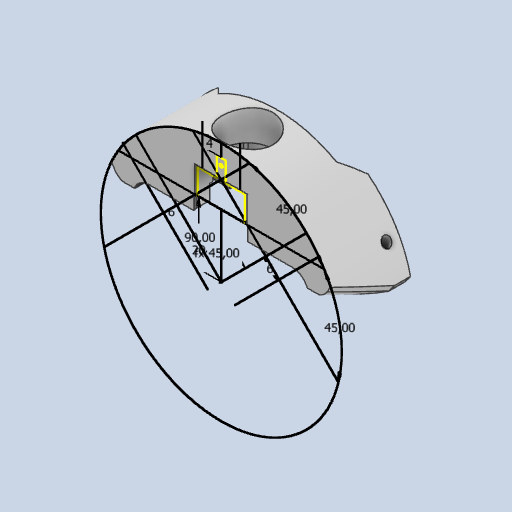
# Autodesk Inventor part: camera_disk
Saved by Autodesk Inventor 2023 (Build 270158000, 158)
## iProperties
Created: 2025-10-11
Part Number: camera_disk
Material: Типовые
Document SubType Name: Modeling
Designer: Andrey
Density: 1 g/cm^3
Appearance: По умолчанию
Author: Andrey
Autodesk Inventor part; units mm, degrees
ref_plane "YZ Plane" through (0, 0, 0) normal (1, 0, 0) x (0, 1, 0)
ref_plane "XZ Plane" through (0, 0, 0) normal (0, 1, 0) x (-1, 0, 0)
ref_plane "XY Plane" through (0, 0, 0) normal (0, 0, 1) x (1, 0, 0)
sketch "Эскиз1" plane through (0, 0, 0) normal (0, 0, 1) x (1, 0, 0)
  line L0 (-15, -8) -> (0, -8) projected
  line L1 (0, 0) -> (0, -8) projected
  line L2 (-6.1, 0) -> (0, 0) projected
  line L3 (-6.1, 0) -> (-6.1, 6.3) projected
  line L4 (-8.9, 6.3) -> (-6.1, 6.3) projected
  line L5 (-8.9, 0) -> (-8.9, 6.3) projected
  line L6 (-15, 0) -> (-8.9, 0) projected
  line L7 (-15, 0) -> (-15, -8) projected
  circle A0 centre (-7.5, 4.1) radius 0.5 projected
  line L8 (-1.5, 13.2534) -> (-1.5, 0.5534)
  line L9 (-13.5, 13.2534) -> (-13.5, 0.5534)
  circle A1 centre (-7.5, -28) radius 38.3
  line L10 (-7.5, -8) -> (-7.5, -28)
  line L11 (-7.5, 6.3) -> (-7.5, 10.3)
  line L12 (-7.5, -28) -> (-34.5822, -0.9178)
  line L13 (-7.5, -28) -> (19.5822, -0.9178)
  line L14 (-11.7426, -32.2426) -> (-38.8248, -5.1605)
  line L15 (-3.2574, -32.2426) -> (23.8248, -5.1605)
  line L16 (25.1633, -8) -> (-40.1633, -8)
  line L17 (1.4543, 9.2386) -> (-44.7386, -36.9543)
  line L18 (29.7386, -36.9543) -> (-16.4543, 9.2386)
  dimension "d0" = 4
  dimension "d1" = 20
  dimension "d2" = 90
  dimension "d3" = 45
  dimension "d4" = 6
  dimension "d5" = 6
  dimension "d13" = 45
  dimension "d17" = 45
  constraints: 22 end point, 5 point on circle, 4 vertical, 2 midpoint, 2 parallel, 1 centre point, 1 coincident, 1 collinear, 1 horizontal, 12 other
  measures "d0" distance of L11.start L11.end
  measures "d1" distance of L10.start L10.end
  measures "d2" angle of L12 L13
  measures "d3" angle of L10 L12
  measures "d4" distance between parallel lines of L12 L14
  measures "d5" distance between parallel lines of L13 L15
sketch "Эскиз2" plane through (0, 0, 0) normal (0, 0, 1) x (1, 0, 0)
  line L0 (-15, -8) -> (0, -8) projected
  line L1 (0, 0) -> (0, -8) projected
  line L2 (-6.1, 0) -> (0, 0) projected
  line L3 (-6.1, 0) -> (-6.1, 6.3) projected
  line L4 (-8.9, 6.3) -> (-6.1, 6.3) projected
  line L5 (-8.9, 0) -> (-8.9, 6.3) projected
  line L6 (-15, 0) -> (-8.9, 0) projected
  line L7 (-15, 0) -> (-15, -8) projected
  circle A0 centre (-7.5, 4.1) radius 0.5 projected
  line L8 (-1.5, 13.2534) -> (-1.5, 0.5534) projected
  line L9 (-13.5, 13.2534) -> (-13.5, 0.5534) projected
  line L10 (4.4, 0) -> (4.4, -8)
  line L11 (-19.4, 0) -> (-19.4, -8)
  line L12 (4.4, -8) -> (-19.4, -8)
  line L13 (-19.4, -8) -> (-19.4, 0)
  line L14 (-19.4, 0) -> (4.4, 0)
  line L15 (4.4, 0) -> (4.4, -8)
  line L16 (0.25, 6.3) -> (0.25, 0)
  line L17 (-15.25, 6.3) -> (-15.25, 0)
  line L18 (-19.7, 0.3) -> (-19.7, -8)
  line L19 (-19.7, 0.3) -> (4.7, 0.3)
  line L20 (4.7, 0.3) -> (4.7, -8)
  line L21 (4.7, -8) -> (-19.7, -8)
  line L22 (-40.1633, -8) -> (25.1633, -8)
  circle A1 centre (-7.5, -28) radius 38.3 projected
  line L23 (0.55, 0) -> (-15.55, 0)
  line L24 (-15.55, 0) -> (-15.55, 10.3)
  line L25 (-15.55, 10.3) -> (0.55, 10.3)
  line L26 (0.55, 10.3) -> (0.55, 0)
  line L27 (-7.5, 6.3) -> (-7.5, 10.3) projected
  line L28 (-25.28, -16.2) -> (10.28, -16.2) projected
  line L29 (10.28, -14.6) -> (10.28, -16.2) projected
  line L30 (-25.28, -14.6) -> (10.28, -14.6) projected
  line L31 (-25.28, -14.6) -> (-25.28, -16.2) projected
  line L32 (10.28, -16.2) -> (-25.28, -16.2)
  line L33 (-25.28, -16.2) -> (-25.28, 10.3)
  line L34 (-25.28, 10.3) -> (10.28, 10.3)
  line L35 (10.28, 10.3) -> (10.28, -16.2)
  point P0 (-25.28, 5.9229)
  point P1 (-25.28, -8)
  point P2 (-15.55, 0.3)
  point P3 (-15.55, 9.4445)
  point P4 (10.28, -8)
  point P5 (10.28, 5.9229)
  point P6 (0.55, 9.4445)
  point P7 (0.55, 0.3)
  dimension "d6" = 0.3
  dimension "d7" = 0.3
  dimension "d8" = 0.3
  constraints: 42 end point, 7 parallel, 4 collinear, 4 vertical, 3 horizontal, 3 perpendicular, 3 point on line, 2 point on circle, 1 midpoint, 9 other
  measures "d6" distance between parallel lines of L11 L18
  measures "d7" distance between parallel lines of L14 L19
  measures "d8" distance between parallel lines of L26 L16
ref_plane "РабПлоскость1" through (-15, -8, -17) normal (0, 0, -1) x (0, 1, 0)
extrude "Выдавливание1" add sketch "Эскиз2" against normal up to surface (17 mm away) contours L22 L33 A1 L24 L19 L18 | L20 L19 L26 A1 L35 L22 | L22 A1 L33 | L35 A1 L22
sketch "Эскиз3" plane through (-40.1633, -8, 0) normal (0, -1, 0) x (1, 0, 0)
  arc A0 (22.6633, -6.6) -> (22.6633, -10.4) centre (22.6633, -8.5) ccw projected
  line L0 (24.1633, -10.4) -> (22.6633, -10.4) projected
  line L1 (22.6633, -6.6) -> (24.1633, -6.6) projected
  arc A1 (42.6633, -10.4) -> (42.6633, -6.6) centre (42.6633, -8.5) ccw projected
  line L2 (42.6633, -10.4) -> (41.1633, -10.4) projected
  line L3 (41.1633, -6.6) -> (42.6633, -6.6) projected
  line L4 (31.2633, 0) -> (31.2633, -0.8775) projected
  arc A2 (31.2633, -0.8775) -> (34.0633, -0.8775) centre (32.6633, -8.5) ccw projected
  line L5 (34.0633, -0.8775) -> (34.0633, 0) projected
  line L6 (34.0633, 0) -> (40.1633, 0) projected
  arc A3 (41.1633, -1) -> (40.1633, 0) centre (40.1633, -1) ccw projected
  line L7 (41.1633, -1) -> (41.1633, -6.6) projected
  line L8 (41.1633, -6.6) -> (42.6633, -6.6) projected
  arc A4 (42.6633, -10.4) -> (42.6633, -6.6) centre (42.6633, -8.5) ccw projected
  line L9 (42.6633, -10.4) -> (41.1633, -10.4) projected
  line L10 (41.1633, -10.4) -> (41.1633, -16) projected
  arc A5 (40.1633, -17) -> (41.1633, -16) centre (40.1633, -16) ccw projected
  line L11 (40.1633, -17) -> (25.1633, -17) projected
  arc A6 (24.1633, -16) -> (25.1633, -17) centre (25.1633, -16) ccw projected
  line L12 (24.1633, -16) -> (24.1633, -10.4) projected
  line L13 (24.1633, -10.4) -> (22.6633, -10.4) projected
  arc A7 (22.6633, -6.6) -> (22.6633, -10.4) centre (22.6633, -8.5) ccw projected
  line L14 (22.6633, -6.6) -> (24.1633, -6.6) projected
  line L15 (24.1633, -6.6) -> (24.1633, -1) projected
  arc A8 (25.1633, 0) -> (24.1633, -1) centre (25.1633, -1) ccw projected
  line L16 (25.1633, 0) -> (31.2633, 0) projected
  circle A9 centre (42.6633, -8.5) radius 0.9 projected
  circle A10 centre (22.6633, -8.5) radius 0.9 projected
  line L17 (23.8633, -10.4) -> (23.8633, -16)
  arc A11 (23.8633, -16) -> (25.1633, -17.3) centre (25.1633, -16) ccw
  line L18 (25.1633, -17.3) -> (40.1633, -17.3)
  arc A12 (40.1633, -17.3) -> (41.4633, -16) centre (40.1633, -16) ccw
  line L19 (41.4633, -16) -> (41.4633, -10.4)
  line L20 (23.8633, -6.6) -> (23.8633, -1)
  arc A13 (25.1633, 0.3) -> (23.8633, -1) centre (25.1633, -1) ccw
  line L21 (25.1633, 0.3) -> (31.5633, 0.3)
  line L22 (31.5633, 0.3) -> (31.5633, -1.1317)
  arc A14 (31.5633, -1.1317) -> (33.7633, -1.1317) centre (32.6633, -8.5) ccw
  line L23 (33.7633, -1.1317) -> (33.7633, 0.3)
  line L24 (33.7633, 0.3) -> (40.1633, 0.3)
  arc A15 (41.4633, -1) -> (40.1633, 0.3) centre (40.1633, -1) ccw
  line L25 (41.4633, -1) -> (41.4633, -6.6)
  arc A16 (22.6633, -6.3) -> (22.6633, -10.7) centre (22.6633, -8.5) ccw
  line L26 (22.6633, -6.3) -> (24.1633, -6.3)
  line L27 (24.1633, -10.7) -> (22.6633, -10.7)
  arc A17 (42.6633, -10.7) -> (42.6633, -6.3) centre (42.6633, -8.5) ccw
  line L28 (42.6633, -10.7) -> (41.1633, -10.7)
  line L29 (41.1633, -6.3) -> (42.6633, -6.3)
  line L30 (20.4633, -17) -> (24.6133, -17) projected
  line L31 (24.6133, 0) -> (24.6133, -17) projected
  line L32 (20.4633, 0) -> (24.6133, 0) projected
  line L33 (20.4633, 0) -> (20.4633, -17) projected
  line L34 (40.7133, -17) -> (44.8633, -17) projected
  line L35 (44.8633, 0) -> (44.8633, -17) projected
  line L36 (40.7133, 0) -> (44.8633, 0) projected
  line L37 (40.7133, 0) -> (40.7133, -17) projected
  point P0 (40.9939, 0)
  point P1 (41.4633, -6.3)
  point P2 (44.8633, -8.5)
  point P3 (41.4633, -10.7)
  point P4 (40.9939, -17)
  point P5 (20.4633, -8.5)
  point P6 (23.8633, -6.3)
  point P7 (24.3326, 0)
  point P8 (24.3326, -17)
  point P9 (23.8633, -10.7)
  point P10 (22.6633, -10.7)
  dimension "d19" = 0.3
  dimension "d20" = 0.3
  dimension "d21" = 0.3
  dimension "d22" = 0.3
  dimension "d23" = 0.3
  dimension "d24" = 0.3
  dimension "d25" = 0.3
  dimension "d26" = 0.3
  constraints: 26 end point, 14 point on circle, 7 centre point, 4 parallel, 12 other
  measures "d19" distance between parallel lines of L12 L17
  measures "d20" distance between parallel lines of L15 L20
  measures "d21" radial gap between concentric circles of A0 A16
  measures "d22" distance between parallel lines of L1 L26
  measures "d23" distance between parallel lines of L0 L27
  measures "d24" radial gap between concentric circles of A1 A17
  measures "d25" distance between parallel lines of L2 L28
  measures "d26" distance between parallel lines of L3 L29
extrude "Выдавливание2" add sketch "Эскиз3" against normal up to surface (8.3 mm away) contours L26 A16 L33 L32 A13 L20 | L17 A11 L30 L33 A16 L27 | A12 L19 L28 A17 L35 L34 | A17 L29 L25 A15 L36 L35
sketch "Эскиз4" plane through (-15.55, 0.3, -17) normal (0, -1, 0) x (1, 0, 0)
  line L0 (6.65, 17) -> (6.65, 16.1225) projected
  arc A0 (6.65, 16.1225) -> (9.45, 16.1225) centre (8.05, 8.5) ccw projected
  line L1 (9.45, 16.1225) -> (9.45, 17) projected
  line L2 (9.45, 17) -> (15.55, 17) projected
  arc A1 (16.55, 16) -> (15.55, 17) centre (15.55, 16) ccw projected
  line L3 (16.55, 16) -> (16.55, 10.4) projected
  line L4 (16.55, 10.4) -> (18.05, 10.4) projected
  arc A2 (18.05, 6.6) -> (18.05, 10.4) centre (18.05, 8.5) ccw projected
  line L5 (18.05, 6.6) -> (16.55, 6.6) projected
  line L6 (16.55, 6.6) -> (16.55, 1) projected
  arc A3 (15.55, 0) -> (16.55, 1) centre (15.55, 1) ccw projected
  line L7 (15.55, 0) -> (0.55, 0) projected
  arc A4 (-0.45, 1) -> (0.55, 0) centre (0.55, 1) ccw projected
  line L8 (-0.45, 1) -> (-0.45, 6.6) projected
  line L9 (-0.45, 6.6) -> (-1.95, 6.6) projected
  arc A5 (-1.95, 10.4) -> (-1.95, 6.6) centre (-1.95, 8.5) ccw projected
  line L10 (-1.95, 10.4) -> (-0.45, 10.4) projected
  line L11 (-0.45, 10.4) -> (-0.45, 16) projected
  arc A6 (0.55, 17) -> (-0.45, 16) centre (0.55, 16) ccw projected
  line L12 (0.55, 17) -> (6.65, 17) projected
  circle A7 centre (18.05, 8.5) radius 0.9 projected
  circle A8 centre (-1.95, 8.5) radius 0.9 projected
  circle A9 centre (8.05, 8.5) radius 7.75
  circle A10 centre (8.05, 8.5) radius 8.05
  line L13 (16.1, 17) -> (16.1, 0) projected
  line L14 (0, 0) -> (16.1, 0)
  line L15 (16.1, 0) -> (16.1, 17)
  line L16 (16.1, 17) -> (0, 17)
  line L17 (0, 17) -> (0, 0)
  point P0 (0, 8.5)
  point P1 (16.1, 8.5)
  point P2 (6.65, 17)
  point P3 (0.55, 17)
  point P4 (0.55, 0)
  point P5 (15.55, 0)
  dimension "d29" = 0.3
  constraints: 8 end point, 2 parallel, 1 centre point, 1 coincident, 1 horizontal, 1 perpendicular, 3 other
extrude "Выдавливание3" add sketch "Эскиз4" against normal up to surface contours L16 L1 A10 L0 | L0 A10 L17 A6 L12 | A6 L17 L16 | L2 A1 L13 A10 L1 | A10 L13 A3 L7 A4 L17 | L16 L13 A1 | A4 L14 L17 | L13 L14 A3 round surface about axis through (-7.5, -28, 0) along (0, 0, -1) radius 38.3 far side no
sketch "Эскиз5" plane through (25.1633, -8, -17) normal (0, -1, 0) x (1, 0, 0)
  circle A0 centre (-47.3933, 13.7) radius 1.4 projected
  circle A1 centre (-17.9333, 13.7) radius 1.4 projected
  line L0 (-40.9183, 16.755) -> (-24.4083, 16.755) projected
  line L1 (-40.9183, 11.421) -> (-40.9183, 16.755) projected
  line L2 (-47.6493, 11.421) -> (-40.9183, 11.421) projected
  line L3 (-48.3867, 11.3072) -> (-47.6493, 11.421) projected
  line L4 (-49.0695, 11.0064) -> (-48.3867, 11.3072) projected
  line L5 (-49.6512, 10.5392) -> (-49.0695, 11.0064) projected
  line L6 (-50.0922, 9.9373) -> (-49.6512, 10.5392) projected
  line L7 (-50.3624, 9.2417) -> (-50.0922, 9.9373) projected
  line L8 (-50.4433, 8.5) -> (-50.3624, 9.2417) projected
  line L9 (-50.3624, 7.7583) -> (-50.4433, 8.5) projected
  line L10 (-50.0922, 7.0627) -> (-50.3624, 7.7583) projected
  line L11 (-49.6512, 6.4608) -> (-50.0922, 7.0627) projected
  line L12 (-49.0695, 5.9936) -> (-49.6512, 6.4608) projected
  line L13 (-48.3867, 5.6928) -> (-49.0695, 5.9936) projected
  line L14 (-47.6493, 5.579) -> (-48.3867, 5.6928) projected
  line L15 (-40.9183, 5.579) -> (-47.6493, 5.579) projected
  line L16 (-40.9183, 0.245) -> (-40.9183, 5.579) projected
  line L17 (-24.4083, 0.245) -> (-40.9183, 0.245) projected
  line L18 (-24.4083, 5.579) -> (-24.4083, 0.245) projected
  line L19 (-17.6773, 5.579) -> (-24.4083, 5.579) projected
  line L20 (-16.9399, 5.6928) -> (-17.6773, 5.579) projected
  line L21 (-16.257, 5.9936) -> (-16.9399, 5.6928) projected
  line L22 (-15.6753, 6.4608) -> (-16.257, 5.9936) projected
  line L23 (-15.2344, 7.0627) -> (-15.6753, 6.4608) projected
  line L24 (-14.9642, 7.7583) -> (-15.2344, 7.0627) projected
  line L25 (-14.8833, 8.5) -> (-14.9642, 7.7583) projected
  line L26 (-14.9642, 9.2417) -> (-14.8833, 8.5) projected
  line L27 (-15.2344, 9.9373) -> (-14.9642, 9.2417) projected
  line L28 (-15.6753, 10.5392) -> (-15.2344, 9.9373) projected
  line L29 (-16.257, 11.0064) -> (-15.6753, 10.5392) projected
  line L30 (-16.9399, 11.3072) -> (-16.257, 11.0064) projected
  line L31 (-17.6773, 11.421) -> (-16.9399, 11.3072) projected
  line L32 (-24.4083, 11.421) -> (-17.6773, 11.421) projected
  line L33 (-24.4083, 16.755) -> (-24.4083, 11.421) projected
  circle A2 centre (-42.6683, 8.505) radius 1.27 projected
  circle A3 centre (-22.6583, 8.505) radius 1.27 projected
  circle A4 centre (-35.9133, 9.695) radius 0.127 projected
  circle A5 centre (-32.7943, 9.512) radius 0.127 projected
  circle A6 centre (-29.2343, 15.993) radius 0.127 projected
  circle A7 centre (-28.5993, 15.993) radius 0.127 projected
  circle A8 centre (-17.4233, 8.5) radius 1.5 projected
  circle A9 centre (-47.9033, 8.5) radius 1.5 projected
  circle A10 centre (-27.4563, 4.69) radius 0.1651 projected
  circle A11 centre (-31.3933, 4.69) radius 0.1651 projected
  circle A12 centre (-26.6943, 6.976) radius 0.2032 projected
  circle A13 centre (-38.1243, 8.754) radius 0.2032 projected
  circle A14 centre (-36.7273, 2.023) radius 0.2032 projected
  circle A15 centre (-39.7753, 16.247) radius 0.2032 projected
  circle A16 centre (-39.1403, 2.023) radius 0.2032 projected
  circle A17 centre (-37.8703, 2.023) radius 0.2032 projected
  circle A18 centre (-35.9145, 15.993) radius 0.127 projected
  circle A19 centre (-32.2823, 15.993) radius 0.127 projected
  circle A20 centre (-27.8373, 15.104) radius 0.127 projected
  circle A21 centre (-38.8863, 15.358) radius 0.1651 projected
  circle A22 centre (-26.6943, 10.786) radius 0.2032 projected
  circle A23 centre (-38.1243, 11.421) radius 0.2032 projected
  circle A24 centre (-29.9133, 15.993) radius 0.127 projected
  circle A25 centre (-38.8863, 14.469) radius 0.1651 projected
  circle A26 centre (-37.8703, 15.358) radius 0.1651 projected
  circle A27 centre (-34.8223, 16.0438) radius 0.127 projected
  circle A28 centre (-29.4133, 9.972) radius 0.127 projected
  circle A29 centre (-31.2155, 8.881) radius 0.127 projected
  circle A30 centre (-29.1073, 8.627) radius 0.127 projected
  circle A31 centre (-35.3303, 8.881) radius 0.127 projected
  circle A32 centre (-30.7863, 16.374) radius 0.127 projected
  circle A33 centre (-34.8731, 5.7314) radius 0.127 projected
  circle A34 centre (-35.6351, 5.7314) radius 0.127 projected
  circle A35 centre (-34.8731, 6.3664) radius 0.127 projected
  circle A36 centre (-33.6031, 8.1444) radius 0.127 projected
  circle A37 centre (-27.3633, 14.445) radius 0.3 projected
  circle A38 centre (-34.1873, 15.993) radius 0.127 projected
  circle A39 centre (-34.3143, 8.881) radius 0.127 projected
  circle A40 centre (-33.6023, 7.357) radius 0.127 projected
  circle A41 centre (-33.5523, 15.993) radius 0.127 projected
  circle A42 centre (-29.9963, 8.119) radius 0.127 projected
  circle A43 centre (-37.7433, 6.341) radius 0.1651 projected
  circle A44 centre (-31.2155, 8.119) radius 0.127 projected
  circle A45 centre (-31.2863, 15.993) radius 0.127 projected
  circle A46 centre (-31.7863, 16.386) radius 0.127 projected
  circle A47 centre (-29.9963, 7.484) radius 0.127 projected
  circle A48 centre (-32.9173, 15.993) radius 0.127 projected
  circle A49 centre (-32.0029, 7.3636) radius 0.127 projected
  circle A50 centre (-37.9633, 14.445) radius 0.3 projected
  line L34 (-41.2183, 11.721) -> (-41.2183, 17.055)
  line L35 (-41.2183, 17.055) -> (-24.1083, 17.055)
  line L36 (-24.1083, 17.055) -> (-24.1083, 11.721)
  line L37 (-24.1083, 11.721) -> (-17.6543, 11.721)
  line L38 (-17.6543, 11.721) -> (-16.8551, 11.5977)
  line L39 (-16.8551, 11.5977) -> (-16.1, 11.265)
  line L40 (-16.1, 11.265) -> (-15.4567, 10.7483)
  line L41 (-15.4567, 10.7483) -> (-14.969, 10.0827)
  line L42 (-14.969, 10.0827) -> (-14.6703, 9.3135)
  line L43 (-14.6703, 9.3135) -> (-14.5815, 8.5)
  line L44 (-14.5815, 8.5) -> (-14.6703, 7.6865)
  line L45 (-14.6703, 7.6865) -> (-14.969, 6.9173)
  line L46 (-14.969, 6.9173) -> (-15.4567, 6.2517)
  line L47 (-15.4567, 6.2517) -> (-16.1, 5.735)
  line L48 (-16.1, 5.735) -> (-16.8551, 5.4023)
  line L49 (-16.8551, 5.4023) -> (-17.6543, 5.279)
  line L50 (-17.6543, 5.279) -> (-24.1083, 5.279)
  line L51 (-24.1083, 5.279) -> (-24.1083, -0.055)
  line L52 (-24.1083, -0.055) -> (-41.2183, -0.055)
  line L53 (-41.2183, -0.055) -> (-41.2183, 5.279)
  line L54 (-41.2183, 5.279) -> (-47.6723, 5.279)
  line L55 (-47.6723, 5.279) -> (-48.4715, 5.4023)
  line L56 (-48.4715, 5.4023) -> (-49.2266, 5.735)
  line L57 (-49.2266, 5.735) -> (-49.8699, 6.2517)
  line L58 (-49.8699, 6.2517) -> (-50.3575, 6.9173)
  line L59 (-50.3575, 6.9173) -> (-50.6563, 7.6865)
  line L60 (-50.6563, 7.6865) -> (-50.7451, 8.5)
  line L61 (-50.7451, 8.5) -> (-50.6563, 9.3135)
  line L62 (-50.6563, 9.3135) -> (-50.3575, 10.0827)
  line L63 (-50.3575, 10.0827) -> (-49.8699, 10.7483)
  line L64 (-49.8699, 10.7483) -> (-49.2266, 11.265)
  line L65 (-49.2266, 11.265) -> (-48.4715, 11.5977)
  line L66 (-48.4715, 11.5977) -> (-47.6723, 11.721)
  line L67 (-47.6723, 11.721) -> (-41.2183, 11.721)
  line L68 (-24.3326, 0) -> (0, 0) projected
  line L69 (0, 17) -> (0, 0) projected
  line L70 (-24.3326, 17) -> (0, 17) projected
  arc A51 (-23.8633, 16) -> (-24.3326, 17) centre (-25.1633, 16) ccw projected
  line L71 (-23.8633, 16) -> (-23.8633, 10.7) projected
  line L72 (-23.8633, 10.7) -> (-22.6633, 10.7) projected
  arc A52 (-22.6633, 6.3) -> (-22.6633, 10.7) centre (-22.6633, 8.5) ccw projected
  line L73 (-22.6633, 6.3) -> (-23.8633, 6.3) projected
  line L74 (-23.8633, 6.3) -> (-23.8633, 1) projected
  arc A53 (-24.3326, 0) -> (-23.8633, 1) centre (-25.1633, 1) ccw projected
  line L75 (-65.3266, 0) -> (-40.9939, 0) projected
  arc A54 (-41.4633, 1) -> (-40.9939, 0) centre (-40.1633, 1) ccw projected
  line L76 (-41.4633, 1) -> (-41.4633, 6.3) projected
  line L77 (-41.4633, 6.3) -> (-42.6633, 6.3) projected
  arc A55 (-42.6633, 10.7) -> (-42.6633, 6.3) centre (-42.6633, 8.5) ccw projected
  line L78 (-42.6633, 10.7) -> (-41.4633, 10.7) projected
  line L79 (-41.4633, 10.7) -> (-41.4633, 16) projected
  arc A56 (-40.9939, 17) -> (-41.4633, 16) centre (-40.1633, 16) ccw projected
  line L80 (-65.3266, 17) -> (-40.9939, 17) projected
  line L81 (-65.3266, 17) -> (-65.3266, 0) projected
  point P0 (-25.1633, 17)
  point P1 (-23.8633, 5.279)
  point P2 (-24.1083, 0.2404)
  point P3 (-24.1083, 0)
  point P4 (-24.1083, 17)
  point P5 (-24.1083, 16.7596)
  point P6 (-23.8633, 11.721)
  point P7 (-41.4633, 11.721)
  point P8 (-41.2183, 16.7596)
  point P9 (-41.2183, 17)
  point P10 (-41.2183, 0)
  point P11 (-41.2183, 0.2404)
  point P12 (-41.4633, 5.279)
  dimension "d32" = 0.3
  constraints: 68 end point, 33 other
  measures "d32" distance between parallel lines of L2 L67
ref_plane "РабПлоскость2" through (6.721, -12.7, -16.201) normal (0, 1, 0) x (0, 0, 1)
extrude "Выдавливание4" add sketch "Эскиз5" along normal up to surface (4.7 mm away) contours L67 L66 L65 L64 L63 L62 L61 L60 L59 L58 L57 L56 L55 L54 L76 A54 L53 L75 L81 L80 L34 A56 L79 | L71 A51 L36 L70 L69 L68 L51 A53 L74 L50 L49 L48 L47 L46 L45 L44 L43 L42 L41 L40 L39 L38 L37
sketch "Эскиз6" plane through (0.8307, 0.3, -17) normal (0, 0, -1) x (-1, 0, 0)
  arc A0 (40.9939, -8.3) -> (-24.3326, -8.3) centre (8.3307, -28.3) ccw projected
  line L0 (-24.3326, -8.3) -> (-24.3326, -13) projected
  line L1 (-0.2243, -13) -> (-24.3326, -13) projected
  line L2 (-0.2243, -8.3) -> (-0.2243, -13) projected
  line L3 (0, -8.3) -> (-0.2243, -8.3) projected
  line L4 (0, -8.3) -> (0, 0) projected
  line L5 (16.6613, 0) -> (0, 0) projected
  line L6 (16.6613, -8.3) -> (16.6613, 0) projected
  line L7 (16.8857, -8.3) -> (16.6613, -8.3) projected
  line L8 (16.8857, -8.3) -> (16.8857, -13) projected
  line L9 (40.9939, -13) -> (16.8857, -13) projected
  line L10 (40.9939, -8.3) -> (40.9939, -13) projected
  line L11 (16.8857, -8.3) -> (16.8857, -13) projected
  line L12 (16.8857, -13) -> (-0.2243, -13)
  line L13 (17.1307, -13) -> (16.8857, -13) projected
  point P0 (0.8307, -0.3)
  constraints: 2 end point, 1 collinear
extrude "Выдавливание5" add sketch "Эскиз6" along normal blind 1
sketch "Эскиз7" plane through (0.8307, 0.3, -18) normal (0, 0, -1) x (-1, 0, 0)
  arc A0 (40.9939, -8.3) -> (-24.3326, -8.3) centre (8.3307, -28.3) ccw projected
  line L0 (-24.3326, -8.3) -> (-24.3326, -13) projected
  line L1 (-24.3326, -13) -> (40.9939, -13) projected
  line L2 (40.9939, -13) -> (40.9939, -8.3) projected
  circle A1 centre (8.3307, -28.3) radius 15.3
  line L3 (-6.9693, -28.3) -> (-29.9693, -28.3)
  circle A2 centre (8.3307, -28.3) radius 38.3
  line L4 (-29.9693, -28.3) -> (46.6307, -28.3)
  line L5 (-9.4493, -14.9) -> (-9.4493, -16.5) projected
  circle A3 centre (8.3307, -28.3) radius 30
  line L6 (-34.6406, -22.3) -> (50.614, -22.3)
  point P0 (0.8307, -0.3)
  point P1 (34.1359, -13)
  point P2 (38.3307, -28.3)
  point P3 (40.9939, -8.3)
  point P4 (-21.6693, -28.3)
  point P5 (-17.4746, -13)
  point P6 (-29.4964, -22.3)
  point P7 (-21.0632, -22.3)
  point P8 (37.7245, -22.3)
  point P9 (46.1578, -22.3)
  dimension "d37" = 60
  dimension "d47" = 6
  constraints: 6 end point, 4 horizontal, 3 coincident, 3 point on circle, 2 centre point, 1 horizontal alignment, 1 point on line, 2 other
  measures "d37" diameter of A3
  measures "d47" distance between parallel lines of L6 L3
extrude "Выдавливание6" add sketch "Эскиз7" against normal up to surface (18 mm away) contours A2 L6 A3 L1 L2 | L0 L1 A3 L6 A2
chamfer "Фаска1" distance 6 angle 45 2 edges at (-36.8939, -22, -9) (21.8939, -22, -9)
fillet "Сопряжение1" radius 5 2 edges at (18.3052, -12.7, -9) (-33.3052, -12.7, -9)
chamfer "Фаска2" distance 6 angle 45 2 edges at (-44.1105, -22, 0) (29.1105, -22, 0)
chamfer "Фаска3" distance 8 angle 45 2 edges at (29.1105, -22, -6) (-44.1105, -22, -6)
chamfer "Фаска4" distance 4 angle 45 2 edges at (29.7625, -19.146, -7.1099) (-44.7625, -19.146, -7.1099)
fillet "Сопряжение2" radius 5 3 edges at (25.5839, -18.5012, -5.5533) (26.967, -21.3176, -14.3807) (-40.5839, -18.5012, -5.5533)
sketch "Эскиз8" plane through (0.8307, 0.3, -18) normal (0, 0, -1) x (-1, 0, 0)
  spline S0 degree 4 poles (43.8453, -22.059) (43.805, -22.1116) (43.7637, -22.1636) (43.7214, -22.215) (43.6781, -22.2658) knots 0 0 0 0 0 1 1 1 1 1 projected
  spline S1 degree 4 poles (45.6494, -19.686) (45.2007, -20.2813) (44.7505, -20.8753) (44.2987, -21.4678) (43.8453, -22.059) knots 0 0 0 0 0 1 1 1 1 1 projected
  arc A0 (45.6494, -19.686) -> (-28.9881, -19.686) centre (8.3307, -28.3) ccw projected
  spline S2 degree 4 poles (-27.184, -22.059) (-27.6374, -21.4678) (-28.0892, -20.8753) (-28.5394, -20.2813) (-28.9881, -19.686) knots 0 0 0 0 0 1 1 1 1 1 projected
  spline S3 degree 4 poles (-27.0167, -22.2658) (-27.06, -22.215) (-27.1023, -22.1636) (-27.1437, -22.1116) (-27.184, -22.059) knots 0 0 0 0 0 1 1 1 1 1 projected
  line L0 (-19.2814, -16.5707) -> (-27.0167, -22.2658) projected
  arc A1 (-19.0049, -15.94) -> (-19.2814, -16.5707) centre (8.3307, -28.3) ccw projected
  arc A2 (-14.4489, -13) -> (-19.0049, -15.94) centre (-14.4489, -18) ccw projected
  line L1 (-14.4489, -13) -> (31.1103, -13) projected
  arc A3 (35.6662, -15.94) -> (31.1103, -13) centre (31.1103, -18) ccw projected
  arc A4 (35.9427, -16.5707) -> (35.6662, -15.94) centre (8.3307, -28.3) ccw projected
  line L2 (43.6781, -22.2658) -> (35.9427, -16.5707) projected
  line L3 (16.8857, -13) -> (31.1103, -13) projected
  line L4 (26.1107, -13) -> (-9.4493, -13)
  line L5 (-9.4493, -13) -> (-9.4493, 17.548)
  line L6 (-9.4493, 17.548) -> (26.1107, 17.548)
  line L7 (26.1107, 17.548) -> (26.1107, -13)
  line L8 (26.1107, -14.9) -> (26.1107, -16.5) projected
  line L9 (-9.4493, -14.9) -> (-9.4493, -16.5) projected
  line L10 (27.1107, -14) -> (-10.4493, -14)
  line L11 (-10.4493, -14) -> (-10.4493, 18.548)
  line L12 (-10.4493, 18.548) -> (27.1107, 18.548)
  line L13 (27.1107, 18.548) -> (27.1107, -14)
  point P0 (0.8307, -0.3)
  point P1 (-10.4493, -13)
  point P2 (-10.4493, 5.0797)
  point P3 (27.1107, 5.0797)
  point P4 (27.1107, -13)
  dimension "d55" = 1
  constraints: 16 end point, 4 parallel, 2 collinear, 2 perpendicular, 1 horizontal, 1 point on line, 7 other
  measures "d55" distance between parallel lines of L7 L13
extrude "Выдавливание7" add sketch "Эскиз8" along normal blind 5 contours S0 L2 A4 A3 L1 L13 A0 S1 | L11 L1 A2 A1 L0 S3 S2 A0
sketch "Эскиз9" plane through (20.112, -16.2707, -23) normal (-0.592884, -0.8052879, 0) x (0.8052879, -0.592884, 0)
  circle A0 centre (1, 4) radius 1.5
  line L0 (0.1222, 22.6569) -> (3.6548, 17.6005) projected
  line L1 (0, 22.7293) -> (0.1222, 22.6569) projected
  line L2 (0, 22.7293) -> (0, 0) projected
  line L3 (9.6057, 0) -> (0, 0) projected
  line L4 (9.6057, 5) -> (9.6057, 0) projected
  point P0 (-25.8426, 23)
  dimension "d58" = 3
  dimension "d59" = 4
  dimension "d60" = 1
  constraints: 1 centre point, 1 other
  measures "d58" diameter of A0
  measures "d59" distance from line of L3 A0.centre
  measures "d60" distance from line of L2 A0.centre
extrude "Выдавливание8" cut sketch "Эскиз9" against normal blind 10
sketch "Эскиз10" plane through (-35.112, -16.2707, -23) normal (0.592884, -0.8052879, 0) x (0.8052879, 0.592884, 0)
  circle A0 centre (-1, 4) radius 1.5
  line L0 (0, 0) -> (-9.6057, 0) projected
  line L1 (0, 0) -> (0, 22.7293) projected
  point P0 (37.9219, 23)
  dimension "d63" = 3
  dimension "d64" = 4
  dimension "d65" = 1
  constraints: 1 centre point
  measures "d63" diameter of A0
  measures "d64" distance from line of L0 A0.centre
  measures "d65" distance from line of L1 A0.centre
extrude "Выдавливание9" cut sketch "Эскиз10" against normal blind 10
chamfer "Фаска5" distance 5 angle 45 2 edges at (-26.28, -3.6602, -23) (11.28, -3.6602, -23)
equation "\"d3\" = 0.5 * d2"
